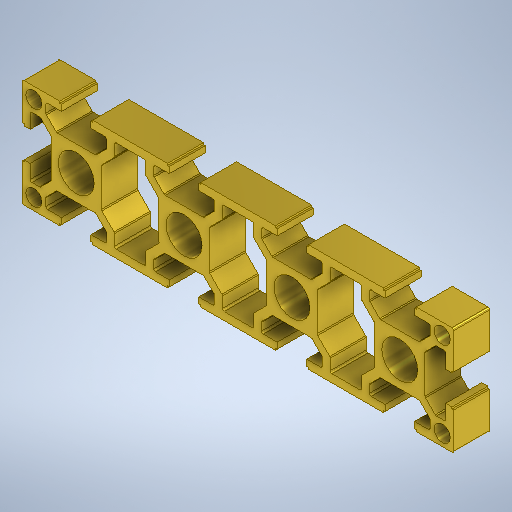
# Autodesk Inventor part: 30×120 10 slots profile_AST03012010
Saved by Autodesk Inventor 2025.2 (Build 292293000, 293)
## iProperties
Created: 2025-04-05
Part Number: 30×120 10 slots profile_AST03012010
Material: Ouro
Document SubType Name: Modeling
Designer: Gustavo Sousa
Density: 19.3 g/cm^3
Appearance: Metal quente 2400F
Author: Gustavo Sousa
Autodesk Inventor part; units mm, degrees
ref_plane "YZ Plane" through (0, 0, 0) normal (1, 0, 0) x (0, 1, 0)
ref_plane "XZ Plane" through (0, 0, 0) normal (0, 1, 0) x (-1, 0, 0)
ref_plane "XY Plane" through (0, 0, 0) normal (0, 0, 1) x (1, 0, 0)
sketch "Esboço2" plane through (0, 0, 0) normal (0, 0, 1) x (1, 0, 0)
  circle A0 centre (-15, 0) radius 5 construction
  line L0 (-15, 15) -> (0, 15) construction
  line L1 (-19.1, 15) -> (-10.9, 15) construction
  line L2 (-15, 0) -> (-15, 5) construction
  line L3 (-15, 0) -> (0, 15) construction
  line L4 (-22, 7) -> (-8, 7) construction
  line L5 (-10.9, 15) -> (-10.9, 12.8) construction
  line L6 (-10.9, 12.8) -> (-6.55, 12.8) construction
  line L7 (-8, 7) -> (-8, -7) construction
  line L8 (-9.5556, 7) -> (-6.55, 10.0056) construction
  line L9 (-6.55, 10.0056) -> (-6.55, 12.8) construction
  line L10 (0, 15) -> (0, 12.8) construction
  line L11 (-4.35, 12.8) -> (0, 12.8) construction
  line L12 (-4.35, 12.8) -> (-4.35, 9.0944) construction
  line L13 (-8, 5.4444) -> (-4.35, 9.0944) construction
  line L14 (-15, 7) -> (-9.5556, 7) construction
  line L15 (-8, 0) -> (-8, 5.4444) construction
  line L16 (-8, 0) -> (-10, 0)
  line L17 (-19.1, 15) -> (-19.1, 12.8) construction
  line L18 (-19.1, 12.8) -> (-23.45, 12.8) construction
  line L19 (-22, 7) -> (-22, -7) construction
  line L20 (-19.1, 15) -> (-30, 15) construction
  line L21 (-30, 15) -> (-15, 0) construction
  line L22 (-23.45, 10.0056) -> (-20.4444, 7) construction
  line L23 (-23.45, 12.8) -> (-23.45, 10.0056) construction
  line L24 (-15, 7) -> (-20.4444, 7) construction
  line L25 (-10.9, 15) -> (0, 15) construction
  line L26 (-25.65, 9.0944) -> (-22, 5.4444) construction
  line L27 (-22, 5.4444) -> (-22, 0) construction
  line L28 (-30, 15) -> (-30, 12.8) construction
  line L29 (-25.65, 9.0944) -> (-25.65, 12.8) construction
  line L30 (-30, 12.8) -> (-25.65, 12.8) construction
  circle A1 centre (-45, 0) radius 5 construction
  line L31 (-30, 15) -> (-45, 0) construction
  line L32 (-52, 7) -> (-38, 7) construction
  line L33 (-49.1, 15) -> (-40.9, 15) construction
  line L34 (-45, 0) -> (-45, 5) construction
  line L35 (-40.9, 15) -> (-30, 15) construction
  line L36 (-40.9, 15) -> (-40.9, 12.8) construction
  line L37 (-39.5556, 7) -> (-36.55, 10.0056) construction
  line L38 (-38, 7) -> (-38, -7) construction
  line L39 (-40.9, 12.8) -> (-36.55, 12.8) construction
  line L40 (-36.55, 12.8) -> (-36.55, 10.0056) construction
  line L41 (-30, 12.8) -> (-34.35, 12.8) construction
  line L42 (-34.35, 12.8) -> (-34.35, 9.0944) construction
  line L43 (-38, 5.4444) -> (-34.35, 9.0944) construction
  line L44 (-38, 5.4444) -> (-38, 0) construction
  line L45 (-39.5556, 7) -> (-45, 7) construction
  line L46 (-52, 7) -> (-52, -7) construction
  line L47 (-45, 15) -> (-60, 15) construction
  line L48 (-60, 15) -> (-45, 0) construction
  line L49 (-49.1, 15) -> (-49.1, 12.8) construction
  line L50 (-49.1, 12.8) -> (-53.45, 12.8) construction
  line L51 (-53.45, 10.0056) -> (-50.4444, 7) construction
  line L52 (-53.45, 10.0056) -> (-53.45, 12.8) construction
  line L53 (-50.4444, 7) -> (-45, 7) construction
  line L54 (-49.1, 15) -> (-60, 15) construction
  line L55 (-52, 0) -> (-50, 0)
  line L56 (-38, 0) -> (-40, 0)
  line L57 (-60, 15) -> (0, 15) construction
  line L58 (-60, 15) -> (-60, -15) construction
  line L59 (-60, 4.1) -> (-60, -4.1) construction
  line L60 (-60, 15) -> (-60, 4.1) construction
  line L61 (-60, 4.1) -> (-57.8, 4.1) construction
  line L62 (-57.8, 8.45) -> (-57.8, 4.1) construction
  line L63 (-55.0056, 8.45) -> (-52, 5.4444) construction
  line L64 (-57.8, 8.45) -> (-55.0056, 8.45) construction
  line L65 (-52, 5.4444) -> (-52, 0) construction
  circle A2 centre (-56.8, 11.8) radius 2.25
  arc A3 (-59.5, 15) -> (-60, 14.5) centre (-59.5, 14.5) ccw
  line L66 (-60, 4.1) -> (-59.5, 4.1) construction
  line L67 (-59.5, 4.1) -> (-59.5, 4.6)
  line L68 (-59.5, 4.6) -> (-60, 4.6)
  line L69 (-60, 4.6) -> (-60, 4.1) construction
  line L70 (-60, 14.5) -> (-60, 4.6)
  line L71 (-59.5, 4.1) -> (-57.8, 4.1)
  arc A4 (-57.3, 8.45) -> (-57.8, 7.95) centre (-57.3, 7.95) ccw
  line L72 (-57.8, 7.95) -> (-57.8, 4.1)
  arc A5 (-54.8592, 8.3036) -> (-55.2127, 8.45) centre (-55.2127, 7.95) ccw
  arc A6 (-52, 5.2373) -> (-52.1464, 5.5908) centre (-52.5, 5.2373) ccw
  line L73 (-57.3, 8.45) -> (-55.2127, 8.45)
  line L74 (-54.8592, 8.3036) -> (-52.1464, 5.5908)
  line L75 (-52, 5.2373) -> (-52, 0)
  line L76 (-49.1, 15) -> (-49.6, 15) construction
  line L77 (-49.6, 15) -> (-49.6, 14.5)
  line L78 (-49.6, 14.5) -> (-49.1, 14.5)
  line L79 (-49.1, 14.5) -> (-49.1, 15) construction
  line L80 (-49.1, 14.5) -> (-49.1, 12.8)
  line L81 (-59.5, 15) -> (-49.6, 15)
  arc A7 (-52.95, 12.8) -> (-53.45, 12.3) centre (-52.95, 12.3) ccw
  arc A8 (-50.5908, 7.1464) -> (-50.2373, 7) centre (-50.2373, 7.5) ccw
  arc A9 (-39.7627, 7) -> (-39.4092, 7.1464) centre (-39.7627, 7.5) ccw
  arc A10 (-36.55, 12.3) -> (-37.05, 12.8) centre (-37.05, 12.3) ccw
  line L82 (-40.9, 15) -> (-40.4, 15) construction
  line L83 (-40.4, 15) -> (-40.4, 14.5)
  line L84 (-40.4, 14.5) -> (-40.9, 14.5)
  line L85 (-40.9, 14.5) -> (-40.9, 15) construction
  line L86 (-40.9, 14.5) -> (-40.9, 12.8)
  line L87 (-40.9, 12.8) -> (-37.05, 12.8)
  arc A11 (-36.6964, 9.8592) -> (-36.55, 10.2127) centre (-37.05, 10.2127) ccw
  line L88 (-36.55, 12.3) -> (-36.55, 10.2127)
  line L89 (-36.6964, 9.8592) -> (-39.4092, 7.1464)
  line L90 (-39.7627, 7) -> (-50.2373, 7)
  arc A12 (-53.45, 10.2127) -> (-53.3036, 9.8592) centre (-52.95, 10.2127) ccw
  line L91 (-49.1, 12.8) -> (-52.95, 12.8)
  line L92 (-53.45, 10.2127) -> (-53.45, 12.3)
  line L93 (-53.3036, 9.8592) -> (-50.5908, 7.1464)
  arc A13 (-37.8536, 5.5908) -> (-38, 5.2373) centre (-37.5, 5.2373) ccw
  line L94 (-38, 5.2373) -> (-38, 0)
  arc A14 (-33.85, 12.8) -> (-34.35, 12.3) centre (-33.85, 12.3) ccw
  arc A15 (-34.4964, 8.9479) -> (-34.35, 9.3015) centre (-34.85, 9.3015) ccw
  line L95 (-37.8536, 5.5908) -> (-34.4964, 8.9479)
  line L96 (-34.35, 9.3015) -> (-34.35, 12.3)
  line L97 (-40.4, 15) -> (-30, 15)
  line L98 (-33.85, 12.8) -> (-30, 12.8)
  arc A16 (-25.65, 12.3) -> (-26.15, 12.8) centre (-26.15, 12.3) ccw
  arc A17 (-25.65, 9.3015) -> (-25.5036, 8.9479) centre (-25.15, 9.3015) ccw
  arc A18 (-22, 5.2373) -> (-22.1464, 5.5908) centre (-22.5, 5.2373) ccw
  line L99 (-30, 12.8) -> (-26.15, 12.8)
  line L100 (-25.65, 12.3) -> (-25.65, 9.3015)
  line L101 (-25.5036, 8.9479) -> (-22.1464, 5.5908)
  line L102 (-22, 5.2373) -> (-22, 0)
  line L103 (-19.1, 15) -> (-19.6, 15) construction
  line L104 (-19.6, 15) -> (-19.6, 14.5)
  line L105 (-19.6, 14.5) -> (-19.1, 14.5)
  line L106 (-19.1, 14.5) -> (-19.1, 15) construction
  line L107 (-30, 15) -> (-19.6, 15)
  line L108 (-19.1, 14.5) -> (-19.1, 12.8)
  arc A19 (-23.45, 10.2127) -> (-23.3036, 9.8592) centre (-22.95, 10.2127) ccw
  arc A20 (-20.5908, 7.1464) -> (-20.2373, 7) centre (-20.2373, 7.5) ccw
  arc A21 (-22.95, 12.8) -> (-23.45, 12.3) centre (-22.95, 12.3) ccw
  arc A22 (-9.7627, 7) -> (-9.4092, 7.1464) centre (-9.7627, 7.5) ccw
  arc A23 (-6.6964, 9.8592) -> (-6.55, 10.2127) centre (-7.05, 10.2127) ccw
  arc A24 (-6.55, 12.3) -> (-7.05, 12.8) centre (-7.05, 12.3) ccw
  line L109 (-10.9, 15) -> (-10.4, 15) construction
  line L110 (-10.4, 15) -> (-10.4, 14.5)
  line L111 (-10.4, 14.5) -> (-10.9, 14.5)
  line L112 (-10.9, 14.5) -> (-10.9, 15) construction
  line L113 (-10.9, 14.5) -> (-10.9, 12.8)
  line L114 (-10.9, 12.8) -> (-7.05, 12.8)
  line L115 (-6.55, 12.3) -> (-6.55, 10.2127)
  line L116 (-6.6964, 9.8592) -> (-9.4092, 7.1464)
  line L117 (-9.7627, 7) -> (-15, 7)
  line L118 (-19.1, 12.8) -> (-22.95, 12.8)
  line L119 (-23.45, 12.3) -> (-23.45, 10.2127)
  line L120 (-23.3036, 9.8592) -> (-20.5908, 7.1464)
  line L121 (-20.2373, 7) -> (-15, 7)
  line L122 (-10.4, 15) -> (0, 15)
  line L123 (0, 15) -> (0, 12.8)
  arc A25 (-7.8536, 5.5908) -> (-8, 5.2373) centre (-7.5, 5.2373) ccw
  arc A26 (-4.4964, 8.9479) -> (-4.35, 9.3015) centre (-4.85, 9.3015) ccw
  arc A27 (-3.85, 12.8) -> (-4.35, 12.3) centre (-3.85, 12.3) ccw
  line L124 (-3.85, 12.8) -> (0, 12.8)
  line L125 (-4.35, 12.3) -> (-4.35, 9.3015)
  line L126 (-4.4964, 8.9479) -> (-7.8536, 5.5908)
  line L127 (-8, 5.2373) -> (-8, 0)
  line L128 (-22, 0) -> (-20, 0)
  arc A28 (-15, 5) -> (-20, 0) centre (-15, 0) ccw
  arc A29 (-10, 0) -> (-15, 5) centre (-15, 0) ccw
  arc A30 (-45, 5) -> (-50, 0) centre (-45, 0) ccw
  arc A31 (-40, 0) -> (-45, 5) centre (-45, 0) ccw
  point P0 (0, 0)
  point P1 (-8.0528, 8.5028)
  point P2 (-60, 0)
  point P3 (-60, 0)
  dimension "d45" = 10
  dimension "d46" = 15
  dimension "d48" = 15
  dimension "d49" = 15
  dimension "d50" = 8.2
  dimension "d51" = 8
  dimension "d55" = 2.2
  dimension "d61" = 1.1
  dimension "d62" = 1.1
  dimension "d64" = 30
  dimension "d75" = 2.2
  dimension "d81" = 4.5
  dimension "d83" = 1.1
  dimension "arco" = 0.5
  dimension "quadrado" = 0.5
  constraints: 258 end point, 64 point on circle, 58 point on line, 51 tangent, 34 equal length, 32 centre point, 30 collinear, 29 vertical, 25 equal radius, 25 horizontal, 19 parallel, 11 midpoint, 10 horizontal alignment, 10 perpendicular, 8 coincident, 5 vertical alignment
  measures "d45" diameter of A0
  measures "d46" distance of point (0, 0) L2.start
  measures "d48" distance of L2.start L0.start
  measures "d49" distance of L0.start L0.end
  measures "d50" distance of L1.start L1.end
  measures "d51" distance between parallel lines of L1 L4
  measures "d55" distance of L6.end L11.start
  measures "d61" distance between parallel lines of L13 L3
  measures "d62" distance from line of point (-8.053, 8.503) L3
  measures "d64" distance of L2.start A1.centre
  measures "d75" distance between parallel lines of L6 L25
  measures "d81" diameter of A2
  measures "d83" distance edge to line of A2 L52
  measures "arco" radius of A3
  measures "quadrado" distance of L67.end L68.end
extrude "Extrusão1" add sketch "Esboço2" along normal mid plane 10
mirror "Espelhar1" about plane through (0, 0, 0) normal (0, 1, 0) of "Extrusão1"
mirror "Espelhar2" about plane through (0, 0, 0) normal (1, 0, 0) of "Extrusão1", "Espelhar1"
